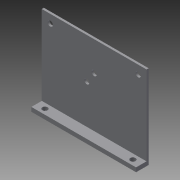
# Autodesk Inventor part: 000110-1
Saved by Autodesk Inventor 2015 (Build 190159000, 159)
## iProperties
Created: 2015-05-13
Part Number: 000110-1
Material: Generic
Document SubType Name: Modeling
Designer: Wesley
Density: 1 g/cm^3
Appearance: Default
Author: Wesley
Autodesk Inventor part; units mm, degrees
ref_plane "YZ Plane" through (0, 0, 0) normal (1, 0, 0) x (0, 1, 0)
ref_plane "XZ Plane" through (0, 0, 0) normal (0, 1, 0) x (-1, 0, 0)
ref_plane "XY Plane" through (0, 0, 0) normal (0, 0, 1) x (1, 0, 0)
sketch "Sketch1" plane through (0, 0, 0) normal (0, 0, 1) x (1, 0, 0)
  line L0 (0, 0) -> (63.5, 0)
  line L1 (63.5, 0) -> (63.5, 50.8)
  line L2 (63.5, 50.8) -> (0, 50.8)
  line L3 (0, 50.8) -> (0, 0)
  dimension "d0" = 50.8
  dimension "d1" = 63.5
  constraints: 8 end point, 2 parallel, 1 horizontal, 1 perpendicular
  measures "d0" distance of L2.end L0.start
  measures "d1" distance of L0.start L0.end
extrude "Extrusion1" add sketch "Sketch1" along normal blind 1.27
sketch "Sketch2" plane through (0, 0, 1.27) normal (0, 0, 1) x (1, 0, 0)
  line L0 (63.5, 0) -> (63.5, 50.8) projected
  line L1 (0, 0) -> (63.5, 0)
  line L2 (63.5, 0) -> (63.5, 2.54)
  line L3 (63.5, 2.54) -> (0, 2.54)
  line L4 (0, 2.54) -> (0, 0)
  dimension "d4" = 2.54
  constraints: 8 end point, 2 parallel, 1 horizontal, 1 perpendicular, 1 point on line
  measures "d4" distance of L3.end L1.start
extrude "Extrusion2" add sketch "Sketch2" along normal blind 6.35
sketch "Sketch3" plane through (0, 0, 1.27) normal (0, 0, 1) x (1, 0, 0)
  line L0 (63.5, 50.8) -> (0, 50.8) projected
  line L1 (63.5, 2.54) -> (63.5, 50.8) projected
  point P0 (0, 0)
  point P1 (31.75, 33.02)
  dimension "d7" = 17.78
  dimension "d8" = 31.75
  measures "d7" distance from line of L0 point (31.75, 33.02)
  measures "d8" distance from line of L1 point (31.75, 33.02)
hole "Hole1" at (31.75, 33.02, 1.27) direction (0, 0, -1) diameter 3.175 depth 25.4 tip angle 118
sketch "Sketch4" plane through (0, 0, 1.27) normal (0, 0, 1) x (1, 0, 0)
  line L0 (0, 50.8) -> (0, 2.54) projected
  line L1 (63.5, 2.54) -> (63.5, 50.8) projected
  line L2 (63.5, 50.8) -> (0, 50.8) projected
  point P0 (0, 0)
  point P1 (5.08, 45.72)
  point P2 (58.42, 45.72)
  dimension "d16" = 5.08
  dimension "d17" = 5.08
  dimension "d18" = 5.08
  dimension "d19" = 5.08
  measures "d16" distance from line of L0 point (5.08, 45.72)
  measures "d17" distance from line of L1 point (58.42, 45.72)
  measures "d18" distance from line of L2 point (58.42, 45.72)
  measures "d19" distance from line of L2 point (5.08, 45.72)
hole "Hole2" at (5.08, 45.72, 1.27) at (58.42, 45.72, 1.27) direction (0, 0, -1) diameter 3.1852 depth 25.4 tip angle 118
sketch "Sketch5" plane through (0, 2.54, 1.27) normal (0, 1, 0) x (1, 0, 0)
  line L0 (63.5, -6.35) -> (0, -6.35) projected
  line L1 (0, 0) -> (0, -6.35) projected
  line L2 (63.5, 0) -> (63.5, -6.35) projected
  point P0 (0, 1.27)
  point P1 (5.08, -3.175)
  point P2 (58.42, -3.175)
  dimension "d27" = 3.175
  dimension "d28" = 5.08
  dimension "d29" = 3.175
  dimension "d30" = 5.08
  measures "d27" distance from line of L0 point (5.08, -3.175)
  measures "d28" distance from line of L1 point (5.08, -3.175)
  measures "d29" distance from line of L0 point (58.42, -3.175)
  measures "d30" distance from line of point (58.42, -3.175) L2
hole "Hole3" at (5.08, 2.54, 4.445) at (58.42, 2.54, 4.445) direction (0, -1, 0) diameter 3.1852 depth 25.4 tip angle 118
sketch "Sketch6" plane through (0, 0, 1.27) normal (0, 0, 1) x (1, 0, 0)
  circle A0 centre (31.75, 33.02) radius 1.5875 construction
  circle A1 centre (31.75, 33.02) radius 3.9751 construction
  circle A2 centre (27.2488, 26.4668) radius 3.9751 construction
  line L0 (63.5, 2.54) -> (0, 2.54) construction
  circle A3 centre (27.2488, 26.4668) radius 1.5875
  line L1 (0, 0) -> (63.5, 0) projected
  dimension "d39" = 7.9502
  dimension "d40" = 7.9502
  dimension "d42" = 3.175
  dimension "d47" = 26.4668
  constraints: 3 centre point, 1 equal radius
  measures "d39" diameter of A2
  measures "d40" diameter of A1
  measures "d42" diameter of A3
  measures "d47" distance from line of L1 A2.centre
extrude "Extrusion3" cut sketch "Sketch6" against normal blind 25.4
body "Solid1"
